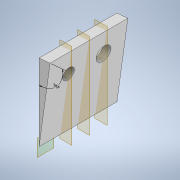
# Autodesk Inventor part: twoPipeCover
Saved by Autodesk Inventor 2021 (Build 250183000, 183)
## iProperties
Created: 2020-07-06
Part Number: twoPipeCover
Material: Generic
Document SubType Name: Modeling
Designer: robst
Density: 1 g/cm^3
Appearance: Default
Author: robst
Autodesk Inventor part; units mm, degrees
ref_plane "YZ Plane" through (0, 0, 0) normal (1, 0, 0) x (0, 1, 0)
ref_plane "XZ Plane" through (0, 0, 0) normal (0, 1, 0) x (-1, 0, 0)
sketch "Sketch1" plane through (0, 0, 0) normal (0, 0, 1) x (1, 0, 0)
  line L0 (0, 0) -> (14.2789, 101.6)
  line L1 (14.2789, 101.6) -> (0, 101.6)
  line L2 (0, 101.6) -> (0, 0)
  dimension "d0" = 101.6
  dimension "d1" = 8
  dimension "d2" = 14.279
  constraints: 6 end point, 1 horizontal, 1 vertical
  measures "d0" distance from line of L0.start L1
  measures "d1" angle of L0 L2
  measures "d2" distance of L0.end L1.end
extrude "Extrusion1" add sketch "Sketch1" along normal mid plane 101.6
ref_plane "Work Plane2" through (0, 0, 42.3872) normal (-1, 0, 0) x (0, 0, 1)
sketch "Sketch7" plane through (0, 0, 0) normal (0, 0, 1) x (1, 0, 0)
  line L0 (0, 101.6) -> (14.2789, 101.6) projected
  line L1 (0, 0) -> (14.2789, 101.6) projected
  line L2 (0, 101.6) -> (0, 0) projected
  line L3 (14.2789, 101.6) -> (0, 101.6) projected
  line L4 (14.2789, 101.6) -> (0, 100.3508)
  line L5 (0, 100.3508) -> (0, 101.6)
  line L6 (0, 101.6) -> (14.2789, 101.6)
  dimension "d27" = 5
  constraints: 6 end point, 1 collinear, 1 perpendicular, 1 point on line
  measures "d27" angle of L0 L4
extrude "Extrusion6" cut sketch "Sketch7" along normal through all both and the other way through all contours L0 L4 L2
sketch "Sketch6" plane through (0, 0, 42.3872) normal (-1, 0, 0) x (0, 0, 1)
  line L0 (-84.1061, 73.66) -> (0, 73.66) construction
  line L1 (0, 101.6) -> (0, 0) construction
  line L2 (-84.7743, 101.6) -> (0, 101.6) construction
  circle A0 centre (-65.2472, 73.66) radius 9.525
  circle A1 centre (-19.5272, 73.66) radius 7.62
  line L3 (-42.3872, 121.92) -> (-42.3872, -20.32) projected
  point P0 (-42.3872, 0)
  dimension "d18" = 27.94
  dimension "d19" = 19.05
  dimension "d20" = 15.24
  dimension "d21" = 22.86
  dimension "d22" = 22.86
  dimension "d23" = 45.72
  constraints: 3 point on line, 2 centre point, 2 end point, 1 horizontal
  measures "d18" distance between parallel lines of L0 L2
  measures "d19" diameter of A0
  measures "d20" diameter of A1
  measures "d21" distance from line of L3 A0.centre
  measures "d22" distance from line of A1.centre L3
  measures "d23" distance of A1.centre A0.centre
extrude "Extrusion5" cut sketch "Sketch6" against normal through all
ref_plane "Work Plane3" through (0, 0, 22.86) normal (0, 0, 1) x (1, 0, 0)
ref_plane "Work Plane4" through (0, 0, -22.86) normal (0, 0, 1) x (1, 0, 0)
sketch "Sketch9" plane through (0, 0, -50.8) normal (-1, 0, 0) x (0, 0, 1)
  line L0 (0, 101.6) -> (0, 0) construction
  line L1 (0, 25.4) -> (100.9997, 25.4) construction
  line L2 (0, 0) -> (101.6, 0) construction
  spline S0 degree 2 poles (31.8744, 22.9804) (31.8744, 21.5602) (30.7937, 19.4143) (29.8984, 18.7042) knots 0 0 0 1 2 2 2
  spline S1 degree 2 poles (29.8984, 18.7042) (28.8177, 17.8551) (26.2551, 17.145) (24.2636, 17.145) knots 0 0 0 1 2 2 2
  line L3 (24.2636, 17.145) -> (16.6529, 17.145)
  line L4 (16.6529, 17.145) -> (16.6529, 36.195)
  line L5 (16.6529, 36.195) -> (23.3683, 36.195)
  spline S2 degree 2 poles (23.3683, 36.195) (25.4678, 36.195) (27.629, 35.8708) (28.5707, 35.3614) knots 0 0 0 1 2 2 2
  spline S3 degree 2 poles (28.5707, 35.3614) (29.605, 34.8211) (30.6085, 32.9685) (30.6085, 31.7644) knots 0 0 0 1 2 2 2
  spline S4 degree 2 poles (30.6085, 31.7644) (30.6085, 30.375) (29.2191, 28.1983) (27.9841, 27.6889) knots 0 0 0 1 2 2 2
  line L6 (27.9841, 27.6889) -> (27.9841, 27.5963)
  spline S5 degree 2 poles (27.9841, 27.5963) (29.7594, 27.2258) (31.8744, 24.9256) (31.8744, 22.9804) knots 0 0 0 1 2 2 2
  spline S6 degree 2 poles (26.9343, 23.0576) (26.9343, 23.953) (26.2242, 24.9564) (25.5141, 25.2189) knots 0 0 0 1 2 2 2
  spline S7 degree 2 poles (25.5141, 25.2189) (25.0818, 25.3887) (23.5535, 25.4196) (22.2876, 25.4196) knots 0 0 0 1 2 2 2
  line L7 (22.2876, 25.4196) -> (21.4077, 25.4196)
  line L8 (21.4077, 25.4196) -> (21.4077, 20.6185)
  line L9 (21.4077, 20.6185) -> (21.6701, 20.6185)
  spline S8 degree 2 poles (21.6701, 20.6185) (23.5226, 20.6185) (24.9429, 20.6648) (25.6839, 20.989) knots 0 0 0 1 2 2 2
  spline S9 degree 2 poles (25.6839, 20.989) (26.3323, 21.2823) (26.9343, 22.3629) (26.9343, 23.0576) knots 0 0 0 1 2 2 2
  spline S10 degree 2 poles (25.7456, 30.8227) (25.7456, 31.2858) (25.2671, 32.2584) (24.7731, 32.4745) knots 0 0 0 1 2 2 2
  spline S11 degree 2 poles (24.7731, 32.4745) (24.3099, 32.6907) (23.0132, 32.7215) (21.7319, 32.7215) knots 0 0 0 1 2 2 2
  line L10 (21.7319, 32.7215) -> (21.4077, 32.7215)
  line L11 (21.4077, 32.7215) -> (21.4077, 28.6769)
  line L12 (21.4077, 28.6769) -> (22.0097, 28.6769)
  spline S12 degree 2 poles (22.0097, 28.6769) (23.2293, 28.6769) (24.2173, 28.7232) (24.7422, 28.9702) knots 0 0 0 1 2 2 2
  spline S13 degree 2 poles (24.7422, 28.9702) (25.3134, 29.2481) (25.7456, 30.1898) (25.7456, 30.8227) knots 0 0 0 1 2 2 2
  line L13 (32.5691, 17.145) -> (39.0065, 36.195)
  line L14 (39.0065, 36.195) -> (44.2245, 36.195)
  line L15 (44.2245, 36.195) -> (50.6619, 17.145)
  line L16 (50.6619, 17.145) -> (45.7373, 17.145)
  line L17 (45.7373, 17.145) -> (44.5486, 21.0353)
  line L18 (44.5486, 21.0353) -> (38.5589, 21.0353)
  line L19 (38.5589, 21.0353) -> (37.3547, 17.145)
  line L20 (37.3547, 17.145) -> (32.5691, 17.145)
  line L21 (43.4989, 24.4933) -> (41.5537, 30.7918)
  line L22 (41.5537, 30.7918) -> (39.5932, 24.4933)
  line L23 (39.5932, 24.4933) -> (43.4989, 24.4933)
  spline S14 degree 2 poles (60.9279, 16.7745) (56.6363, 16.7745) (51.6036, 21.9615) (51.6036, 26.6546) knots 0 0 0 1 2 2 2
  spline S15 degree 2 poles (51.6036, 26.6546) (51.6036, 31.1778) (56.6517, 36.5655) (60.9434, 36.5655) knots 0 0 0 1 2 2 2
  spline S16 degree 2 poles (60.9434, 36.5655) (62.0703, 36.5655) (63.892, 36.3031) (64.7256, 36.0869) knots 0 0 0 1 2 2 2
  spline S17 degree 2 poles (64.7256, 36.0869) (65.374, 35.8862) (66.9023, 35.2224) (67.3809, 34.9754) knots 0 0 0 1 2 2 2
  line L24 (67.3809, 34.9754) -> (67.3809, 30.4368)
  line L25 (67.3809, 30.4368) -> (66.9023, 30.4368)
  spline S18 degree 2 poles (66.9023, 30.4368) (66.5472, 30.7455) (65.4975, 31.61) (64.8336, 32.0114) knots 0 0 0 1 2 2 2
  spline S19 degree 2 poles (64.8336, 32.0114) (64.1698, 32.4282) (62.5798, 32.9994) (61.6998, 32.9994) knots 0 0 0 1 2 2 2
  spline S20 degree 2 poles (61.6998, 32.9994) (60.6655, 32.9994) (58.9519, 32.351) (58.1646, 31.5328) knots 0 0 0 1 2 2 2
  spline S21 degree 2 poles (58.1646, 31.5328) (57.4545, 30.8073) (56.5437, 28.3218) (56.5437, 26.6391) knots 0 0 0 1 2 2 2
  spline S22 degree 2 poles (56.5437, 26.6391) (56.5437, 24.8638) (57.4853, 22.4401) (58.2572, 21.6991) knots 0 0 0 1 2 2 2
  spline S23 degree 2 poles (58.2572, 21.6991) (58.9982, 20.9735) (60.8199, 20.3406) (61.7307, 20.3406) knots 0 0 0 1 2 2 2
  spline S24 degree 2 poles (61.7307, 20.3406) (62.6724, 20.3406) (64.386, 20.9735) (64.9726, 21.3595) knots 0 0 0 1 2 2 2
  spline S25 degree 2 poles (64.9726, 21.3595) (65.621, 21.7454) (66.5935, 22.5636) (66.9486, 22.8878) knots 0 0 0 1 2 2 2
  line L26 (66.9486, 22.8878) -> (67.3809, 22.8878)
  line L27 (67.3809, 22.8878) -> (67.3809, 18.4109)
  spline S26 degree 2 poles (67.3809, 18.4109) (66.856, 18.1639) (65.482, 17.5464) (64.741, 17.3303) knots 0 0 0 1 2 2 2
  spline S27 degree 2 poles (64.741, 17.3303) (63.8456, 17.0524) (62.2864, 16.7745) (60.9279, 16.7745) knots 0 0 0 1 2 2 2
  line L28 (86.894, 17.145) -> (81.1049, 17.145)
  line L29 (81.1049, 17.145) -> (75.9333, 24.8792)
  line L30 (75.9333, 24.8792) -> (74.9916, 23.5825)
  line L31 (74.9916, 23.5825) -> (74.9916, 17.145)
  line L32 (74.9916, 17.145) -> (70.2059, 17.145)
  line L33 (70.2059, 17.145) -> (70.2059, 36.195)
  line L34 (70.2059, 36.195) -> (74.9916, 36.195)
  line L35 (74.9916, 36.195) -> (74.9916, 27.6889)
  line L36 (74.9916, 27.6889) -> (81.1049, 36.195)
  line L37 (81.1049, 36.195) -> (86.6161, 36.195)
  line L38 (86.6161, 36.195) -> (79.8236, 27.3493)
  line L39 (79.8236, 27.3493) -> (86.894, 17.145)
  point P0 (50.8, 0)
  dimension "d35" = 25.4
  constraints: 2 end point, 2 horizontal, 1 point on line
  measures "d35" distance between parallel lines of L1 L2
extrude "Extrusion7" cut sketch "Sketch9" against normal blind 2.032
body "Solid1"
